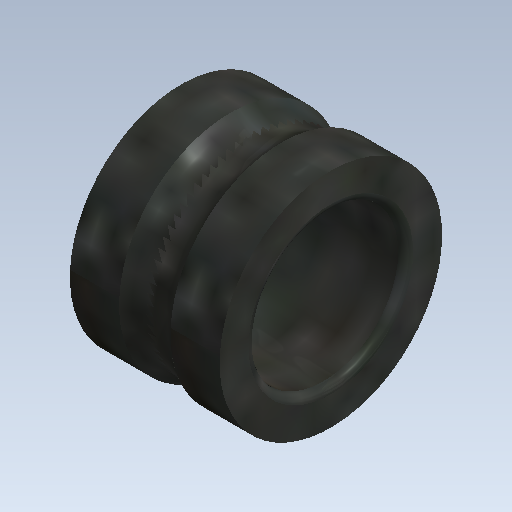
# Autodesk Inventor part: 606 Inner Ring
Saved by Autodesk Inventor 2021 (Build 250183000, 183)
## iProperties
Part Number: 606 Inner Ring
Material: Steel
Catalog Web Link: www.cadenas.de
Description: open_type_IR-
Vendor: NSK_RB
Document SubType Name: Modeling
Designer: partserver
Manufacturer: NSK_RB
Mass: 1.49816 g
Surface Area: 3.46168 cm^2
Volume: 0.190848 cm^3
Density: 7.85 g/cm^3
Appearance: Plate
Category: PARTsolutions
Company: NSK_RB
PSOL_IDENT_0: {$CADENAS_DATA\23d-libs\nsk_rb\roller_bearings\deep_groove_bb\exstra_small_miniatur_bb\metric_design
PSOL_IDENT_1: \open_type_ir_1.prj},176 {VTYP=3D},{NB=606 Inner Ring},{LINA=606 Inner Ring},{NN=open_type_IR},{DATE=
PSOL_IDENT_2: 10.04.2020 04:57:44},{GEOMDATE=04.01.2008 00:00:00},{VERSION=},{LINEID=1680},{WBVAR=},{WBNUMERIC=}
PSOL_IDENT_3: {NB=606 Inner Ring},{LINA=606 Inner Ring},{KT=DUMMY},{IDNR=},{STAN=Standard},{ORDER=606},{SD=6.0},{X=
PSOL_IDENT_4: 6.0},{DI1=8.92},{SDE1=13.75},{D=17},{DD=17},{B=6.0},{B1=0.0},{R=0.30},{R1=0.00},{CR1=2260},{COR1=835
PSOL_IDENT_5: },{CR2=231},{COR2=85.0},{LG=38000},{LO=45000},{DA=8.0},{DB=0.0},{DA1=15.0},{DB1=0.0},{RA=0.30},{RB=0
PSOL_IDENT_6: .00},{MASS=5.97},{SC=1},{N=8}
NB: 606 Inner Ring
NN: open_type_IR
NBSYN: $ORDER. Inner Ring
LINA: 606 Inner Ring
CATALOG: NSK Rolling Bearing
STAN: Standard
ORDER: 606
SD: 6
X: 6
DI1: 8.92
SDE1: 13.75
D: 17
DD: 17
B: 6
B1: 0
R: 0.3
R1: 0
CR1: 2260
COR1: 835
CR2: 231
COR2: 85
LG: 38000
LO: 45000
DA: 8
DB: 0
DA1: 15
DB1: 0
RA: 0.3
RB: 0
MASS: 5.97
SC: 1
SUPPLIER: NSK_RB
ARTICLENO: 606 Inner Ring
BOMINFO: 606 Inner Ring
CREATOR: CADENAS GmbH
Title: 606 Inner Ring
Author: Cadenas PARTsolutions
Autodesk Inventor part; units mm, degrees
sketch "Sketch_1" plane through (0, 0, 0) normal (0, 0, 1) x (1, 0, 0)
  line L0 (6, 0) -> (0, 0)
  arc A0 (0, 3.3) -> (0.3, 3) centre (0.3, 3.3) ccw
  line L1 (0.3, 3) -> (5.7, 3)
  arc A1 (5.7, 3) -> (6, 3.3) centre (5.7, 3.3) ccw
  line L2 (6, 3.3) -> (6, 4.46)
  line L3 (6, 4.46) -> (4.0288, 4.46)
  arc A2 (1.9712, 4.46) -> (4.0288, 4.46) centre (3, 5.75) ccw
  line L4 (1.9712, 4.46) -> (0, 4.46)
  line L5 (0, 4.46) -> (0, 3.3)
  constraints: 12 end point, 6 point on circle, 3 centre point
revolve "Revolution1" add sketch "Sketch_1" angle 360 about axis through (6, 0, 0) along (1, 0, 0)
ref_plane "ip_op_ir_1_1_XY" through (3, 5.75, 0) normal (1, 0, 0) x (0, 0, -1)
ref_plane "ip_op_ir_1_1_YZ" through (3, 5.75, 0) normal (0, 0, -1) x (0, 1, 0)
ref_plane "ip_op_ir_1_1_ZX" through (3, 5.75, 0) normal (0, 1, 0) x (1, 0, 0)
ref_plane "ip_op_ir_1_2_XY" through (3, 4.0659, 4.0659) normal (1, 0, 0) x (0, 0, -1)
ref_plane "ip_op_ir_1_2_YZ" through (3, 4.0659, 4.0659) normal (0, 0, -1) x (0, 1, 0)
ref_plane "ip_op_ir_1_2_ZX" through (3, 4.0659, 4.0659) normal (0, 1, 0) x (1, 0, 0)
ref_plane "ip_op_ir_1_3_XY" through (3, 0, 5.75) normal (1, 0, 0) x (0, 0, -1)
ref_plane "ip_op_ir_1_3_YZ" through (3, 0, 5.75) normal (0, 0, -1) x (0, 1, 0)
ref_plane "ip_op_ir_1_3_ZX" through (3, 0, 5.75) normal (0, 1, 0) x (1, 0, 0)
ref_plane "ip_op_ir_1_4_XY" through (3, -4.0659, 4.0659) normal (1, 0, 0) x (0, 0, -1)
ref_plane "ip_op_ir_1_4_YZ" through (3, -4.0659, 4.0659) normal (0, 0, -1) x (0, 1, 0)
ref_plane "ip_op_ir_1_4_ZX" through (3, -4.0659, 4.0659) normal (0, 1, 0) x (1, 0, 0)
ref_plane "ip_op_ir_1_5_XY" through (3, -5.75, 0) normal (1, 0, 0) x (0, 0, -1)
ref_plane "ip_op_ir_1_5_YZ" through (3, -5.75, 0) normal (0, 0, -1) x (0, 1, 0)
ref_plane "ip_op_ir_1_5_ZX" through (3, -5.75, 0) normal (0, 1, 0) x (1, 0, 0)
ref_plane "ip_op_ir_1_6_XY" through (3, -4.0659, -4.0659) normal (1, 0, 0) x (0, 0, -1)
ref_plane "ip_op_ir_1_6_YZ" through (3, -4.0659, -4.0659) normal (0, 0, -1) x (0, 1, 0)
ref_plane "ip_op_ir_1_6_ZX" through (3, -4.0659, -4.0659) normal (0, 1, 0) x (1, 0, 0)
ref_plane "ip_op_ir_1_7_XY" through (3, 0, -5.75) normal (1, 0, 0) x (0, 0, -1)
ref_plane "ip_op_ir_1_7_YZ" through (3, 0, -5.75) normal (0, 0, -1) x (0, 1, 0)
ref_plane "ip_op_ir_1_7_ZX" through (3, 0, -5.75) normal (0, 1, 0) x (1, 0, 0)
ref_plane "ip_op_ir_1_8_XY" through (3, 4.0659, -4.0659) normal (1, 0, 0) x (0, 0, -1)
ref_plane "ip_op_ir_1_8_YZ" through (3, 4.0659, -4.0659) normal (0, 0, -1) x (0, 1, 0)
ref_plane "ip_op_ir_1_8_ZX" through (3, 4.0659, -4.0659) normal (0, 1, 0) x (1, 0, 0)
ref_plane "ip_op_ir_1a_XY" through (0, 0, 0) normal (1, 0, 0) x (0, 0, -1)
ref_plane "ip_op_ir_1a_YZ" through (0, 0, 0) normal (0, 0, -1) x (0, 1, 0)
ref_plane "ip_op_ir_1a_ZX" through (0, 0, 0) normal (0, 1, 0) x (1, 0, 0)
body "Solid1"
